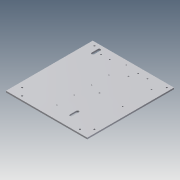
# Autodesk Inventor part: NewBackPlate
Saved by Autodesk Inventor 2014 (Build 180170000, 170)
## iProperties
Created: 2014-08-10
Part Number: NewBackPlate
Material: Generic
Document SubType Name: Modeling
Designer: Peele
Density: 1 g/cm^3
Appearance: White
Author: Peele
Autodesk Inventor part; units mm, degrees
ref_plane "YZ Plane" through (0, 0, 0) normal (1, 0, 0) x (0, 1, 0)
ref_plane "XZ Plane" through (0, 0, 0) normal (0, 1, 0) x (-1, 0, 0)
ref_plane "XY Plane" through (0, 0, 0) normal (0, 0, 1) x (1, 0, 0)
sketch "Sketch1" plane through (0, 0, 0) normal (0, 0, 1) x (1, 0, 0)
  line L0 (-140.5, -150) -> (140.5, -150)
  line L1 (140.5, -150) -> (140.5, 150)
  line L2 (140.5, 150) -> (-140.5, 150)
  line L3 (-140.5, 150) -> (-140.5, -150)
  line L4 (-140.5, -150) -> (140.5, 150) construction
  line L5 (140.5, -150) -> (-140.5, 150) construction
  point P0 (0, 0)
  dimension "d0" = 300
  dimension "d1" = 281
  constraints: 12 end point, 2 midpoint, 2 parallel, 1 horizontal, 1 perpendicular
  measures "d0" distance of L2.end L0.start
  measures "d1" distance of L1.end L2.end
extrude "Extrusion1" add sketch "Sketch1" along normal blind 5
sketch "Sketch5" plane through (0, 0, 5) normal (0, 0, 1) x (1, 0, 0)
  line L0 (-140.5, -150) -> (140.5, -150) projected
  line L1 (140.5, -150) -> (140.5, 150) projected
  line L2 (140.5, 150) -> (-140.5, 150) projected
  line L3 (-140.5, 150) -> (-140.5, -150) projected
  line L4 (-122, -112.5) -> (128, -112.5) construction
  line L5 (128, -112.5) -> (128, 137.5) construction
  line L6 (128, 137.5) -> (-122, 137.5) construction
  line L7 (-122, 137.5) -> (-122, -112.5) construction
  line L8 (-122, -112.5) -> (128, 137.5) construction
  line L9 (128, -112.5) -> (-122, 137.5) construction
  circle A0 centre (-122, 137.5) radius 2.7
  circle A1 centre (128, 137.5) radius 2.7
  circle A2 centre (128, -112.5) radius 2.7
  circle A3 centre (-122, -112.5) radius 2.7
  circle A4 centre (-97, -137.5) radius 2.7
  circle A5 centre (103, -137.5) radius 2.7
  point P0 (0, 0)
  point P1 (3, 12.5)
  dimension "d34" = 18.5
  dimension "d35" = 37.5
  dimension "d36" = 12.5
  dimension "d37" = 5.4
  dimension "d38" = 12.5
  dimension "d39" = 37.5
  dimension "d40" = 43.5
  dimension "d83" = 12.5
  constraints: 12 end point, 6 centre point, 5 equal radius, 4 coincident, 2 midpoint, 2 parallel, 1 horizontal, 1 horizontal alignment, 1 perpendicular
  measures "d34" distance between parallel lines of L3 L7
  measures "d35" distance between parallel lines of L4 L0
  measures "d36" distance between parallel lines of L2 L6
  measures "d37" diameter of A1
  measures "d38" distance from line of A5.centre L0
  measures "d39" distance from line of A5.centre L1
  measures "d40" distance from line of L3 A4.centre
  measures "d83" distance between parallel lines of L5 L1
extrude "Extrusion5" cut sketch "Sketch5" against normal through all contours A0 | A1 | A2 | A3 | A4 | A5
sketch "Sketch6" plane through (0, 0, 5) normal (0, 0, 1) x (1, 0, 0)
  line L0 (-140.5, -150) -> (140.5, -150) projected
  line L1 (140.5, -150) -> (140.5, 150) projected
  line L2 (-140.5, 150) -> (-140.5, -150) projected
  line L3 (-17, -110) -> (-2, -110) construction
  line L4 (-2, -110) -> (-2, 140) construction
  line L5 (-2, 140) -> (-17, 140) construction
  line L6 (-17, 140) -> (-17, -110) construction
  line L7 (-17, -110) -> (-2, 140) construction
  line L8 (-2, -110) -> (-17, 140) construction
  circle A0 centre (-9.5, 15) radius 1.6
  circle A1 centre (-9.5, 75) radius 1.6
  circle A2 centre (-9.5, 135) radius 1.6
  circle A3 centre (-9.5, -45) radius 1.6
  circle A4 centre (-9.5, -105) radius 1.6
  line L9 (-9.5, -105) -> (-9.5, -45) construction
  line L10 (-9.5, -45) -> (-9.5, 15) construction
  line L11 (-9.5, 15) -> (-9.5, 75) construction
  line L12 (-9.5, 75) -> (-9.5, 135) construction
  line L13 (115.5, -150) -> (-134.5, -150) construction
  line L14 (-134.5, -150) -> (-134.5, 62.3779) construction
  line L15 (-134.5, 62.3779) -> (115.5, 62.3779) construction
  line L16 (115.5, 62.3779) -> (115.5, -150) construction
  line L17 (-9.5, 62.3779) -> (-9.5, 15) construction
  point P0 (0, 0)
  dimension "d43" = 250
  dimension "d44" = 15
  dimension "d45" = 60
  dimension "d46" = 3.2
  dimension "d47" = 6
  dimension "d48" = 25
  dimension "d49" = 40
  constraints: 30 end point, 6 parallel, 5 centre point, 4 collinear, 4 equal radius, 3 midpoint, 2 horizontal, 2 perpendicular, 2 vertical, 1 coincident, 1 point on line
  measures "d43" distance of L3.end L4.end
  measures "d44" distance of L4.end L5.end
  measures "d45" distance of L9.start L9.end
  measures "d46" diameter of A4
  measures "d47" distance between parallel lines of L2 L14
  measures "d48" distance between parallel lines of L1 L16
  measures "d49" distance between parallel lines of L3 L13
extrude "Extrusion6" cut sketch "Sketch6" against normal through all
sketch "Sketch7" plane through (0, 0, 0) normal (0, 0, -1) x (-1, 0, 0)
  circle A0 centre (9.5, 135) radius 1.6 projected
  circle A1 centre (122, 137.5) radius 2.7 projected
  circle A2 centre (-128, 137.5) radius 2.7 projected
  line L0 (140.5, -150) -> (-140.5, -150) projected
  line L1 (140.5, 150) -> (140.5, -150) projected
  line L2 (-140.5, 150) -> (140.5, 150) projected
  line L3 (-140.5, -150) -> (-140.5, 150) projected
  line L4 (-53, -125) -> (-103, -125) construction
  line L5 (-103, -125) -> (-103, -74) construction
  line L6 (-103, -74) -> (-53, -74) construction
  line L7 (-53, -74) -> (-53, -125) construction
  line L8 (94.5, 150) -> (44.5, 150) construction
  line L9 (44.5, 150) -> (44.5, 96) construction
  line L10 (44.5, 96) -> (94.5, 96) construction
  line L11 (94.5, 96) -> (94.5, 150) construction
  circle A3 centre (54.5, 123) radius 2.2
  circle A4 centre (84.5, 123) radius 2.2
  line L12 (-45.5, -88.5) -> (-45.5, -110.5) construction
  line L13 (-50, -88.5) -> (-50, -110.5)
  line L14 (-41, -110.5) -> (-41, -88.5)
  arc A5 (-41, -88.5) -> (-50, -88.5) centre (-45.5, -88.5) ccw
  arc A6 (-50, -110.5) -> (-41, -110.5) centre (-45.5, -110.5) ccw
  line L15 (-45.5, -99.5) -> (-103, -99.5) construction
  line L16 (69.5, 96) -> (69.5, 144) construction
  line L17 (102, 134) -> (102, 112) construction
  line L18 (97.5, 134) -> (97.5, 112)
  line L19 (106.5, 112) -> (106.5, 134)
  arc A7 (106.5, 134) -> (97.5, 134) centre (102, 134) ccw
  arc A8 (97.5, 112) -> (106.5, 112) centre (102, 112) ccw
  line L20 (-73.3625, 150) -> (-30.5, 150) construction
  line L21 (-30.5, 150) -> (-30.5, 124.9969) construction
  line L22 (-30.5, 124.9969) -> (-73.3625, 124.9969) construction
  line L23 (-73.3625, 124.9969) -> (-73.3625, 150) construction
  circle A9 centre (-67.8063, 130.5531) radius 2.286
  circle A10 centre (-36.0563, 130.5531) radius 2.286
  line L24 (-108, 4.9969) -> (-28, 4.9969) construction
  line L25 (-28, 4.9969) -> (-28, 104.9969) construction
  line L26 (-28, 104.9969) -> (-108, 104.9969) construction
  line L27 (-108, 104.9969) -> (-108, 4.9969) construction
  line L28 (-108, 4.9969) -> (-28, 104.9969) construction
  line L29 (-28, 4.9969) -> (-108, 104.9969) construction
  circle A11 centre (-108, 104.9969) radius 2.2
  circle A12 centre (-28, 104.9969) radius 2.2
  circle A13 centre (-28, 4.9969) radius 2.2
  circle A14 centre (-108, 4.9969) radius 2.2
  point P0 (0, 0)
  point P1 (102, 123)
  point P2 (-68, 54.9969)
  dimension "d52" = 50
  dimension "d53" = 51
  dimension "d54" = 25
  dimension "d55" = 54
  dimension "d56" = 50
  dimension "d57" = 30
  dimension "d58" = 4.4
  dimension "d59" = 10
  dimension "d60" = 27
  dimension "d61" = 37.5
  dimension "d62" = 22
  dimension "d63" = 9
  dimension "d64" = 3
  dimension "d65" = 60
  dimension "d66" = 3
  dimension "d67" = 15.5
  dimension "d68" = 31.75
  dimension "d69" = 42.8625
  dimension "d70" = 5.5563
  dimension "d71" = 25.0031
  dimension "d72" = 5.5563
  dimension "d73" = 4.572
  dimension "d74" = 35
  dimension "d75" = 40
  dimension "d76" = 100
  dimension "d77" = 80
  dimension "d78" = 4.4
  dimension "d79" = 20
  dimension "d80" = 20
  constraints: 56 end point, 13 parallel, 12 centre point, 8 point on circle, 8 tangent, 6 equal radius, 6 midpoint, 5 horizontal, 5 perpendicular, 4 coincident, 3 horizontal alignment, 3 point on line
  measures "d52" distance of L5.end L6.end
  measures "d53" distance of L6.end L4.start
  measures "d54" distance between parallel lines of L0 L4
  measures "d55" distance of L10.end L8.start
  measures "d56" distance of L9.end L10.end
  measures "d57" distance of A3.centre A4.centre
  measures "d58" diameter of A3
  measures "d59" distance from line of A4.centre L11
  measures "d60" distance from line of L8 A4.centre
  measures "d61" distance between parallel lines of L3 L5
  measures "d62" distance of L12.start L12.end
  measures "d63" distance between parallel lines of L13 L14
  measures "d64" distance between parallel lines of L7 L13
  measures "d65" distance from line of A0.centre L16
  measures "d66" distance between parallel lines of L11 L18
  measures "d67" distance from line of L19 A1.centre
  measures "d68" distance of A9.centre A10.centre
  measures "d69" distance of L21.end L22.end
  measures "d70" distance from line of A10.centre L22
  measures "d71" distance of L22.end L20.start
  measures "d72" distance from line of A9.centre L23
  measures "d73" diameter of A10
  measures "d74" distance from line of A0.centre L9
  measures "d75" distance from line of L21 A0.centre
  measures "d76" distance of L26.end L24.start
  measures "d77" distance of L25.end L26.end
  measures "d78" diameter of A11
  measures "d79" distance from line of A2.centre L27
  measures "d80" distance between parallel lines of L26 L22
extrude "Extrusion7" cut sketch "Sketch7" against normal through all contours A3 | A4 | A5 L14 A6 L13 | A7 L19 A8 L18 | A9 | A10 | A11 | A12 | A13 | A14
equation "\"d59\" = -0.5 * d57 + 0.5 * d56"
equation "\"d60\" = 0.5 * d55"
equation "\"d72\" = -0.5 * d68 + 0.5 * d69"
body "Solid1"
